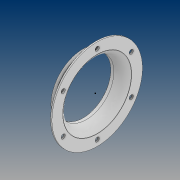
# Autodesk Inventor part: kelifos 3
Saved by Autodesk Inventor 2021 (Build 250183000, 183)
## iProperties
Created: 2021-01-08
Part Number: kelifos 3
Material: Generic
Document SubType Name: Sheet Metal
Designer: Διογενης Τσιχλακης
Density: 1 g/cm^3
Sheet Metal Rule: Default_mm
Appearance: Default
Author: Διογενης Τσιχλακης
Autodesk Inventor part; units mm, degrees
ref_plane "YZ Plane" through (0, 0, 0) normal (1, 0, 0) x (0, 1, 0)
ref_plane "XZ Plane" through (0, 0, 0) normal (0, 1, 0) x (-1, 0, 0)
ref_plane "XY Plane" through (0, 0, 0) normal (0, 0, 1) x (1, 0, 0)
sketch "Sketch1" plane through (0, 0, 0) normal (1, 0, 0) x (0, 1, 0)
  circle A0 centre (0, 0) radius 268
  circle A1 centre (0, 0) radius 232.5
  circle A2 centre (0, 0) radius 203.25
  circle A3 centre (232.5, 0) radius 12.5
  circle A4 centre (116.25, 201.3509) radius 12.5
  circle A5 centre (-116.25, 201.3509) radius 12.5
  circle A6 centre (-232.5, 0) radius 12.5
  circle A7 centre (-116.25, -201.3509) radius 12.5
  circle A8 centre (116.25, -201.3509) radius 12.5
  dimension "d1" = 465
  dimension "d0" = 536
  dimension "d2" = 406.5
  dimension "d3" = 25
  dimension "d52" = 360
  constraints: 8 centre point, 3 coincident, 1 horizontal alignment, 15 other
  measures "d0" diameter of A0
  measures "d2" diameter of A2
  measures "d3" diameter of A3
extrude "Extrusion1" add sketch "Sketch1" along normal blind 10 contours A0 | A3 A1 A8 A7 A6 A5 A4
sketch "Sketch2" plane through (0, 0, 0) normal (0, 1, 0) x (-1, 0, 0)
  line L0 (-10, 203.25) -> (0, 203.25) projected
  line L1 (-10, 203.25) -> (0, 203.25)
  line L2 (-10, 203.25) -> (-10, 193.1351)
  line L3 (-10, 188.8509) -> (-10, 213.8509) projected
  line L4 (0, 268) -> (0, -268) projected
  line L5 (0, 0) -> (70, 0)
  line L6 (70, 163.9189) -> (70, 0)
  line L7 (70, 0) -> (55, 0)
  line L8 (55, 163.9189) -> (55, 188.9189)
  line L9 (-10, -203.25) -> (-10, 203.25) projected
  line L10 (55, 163.9189) -> (55, 173.9189)
  line L11 (55, 188.9189) -> (65, 188.9189)
  line L12 (55, 163.9189) -> (65, 163.9189)
  line L13 (65, 163.9189) -> (70, 163.9189)
  line L14 (70, 188.9189) -> (65, 188.9189)
  line L15 (70, 163.9189) -> (75, 163.9189)
  line L16 (75, 163.9189) -> (75, 188.9189)
  line L17 (75, 188.9189) -> (70, 188.9189)
  line L18 (-10, 193.1351) -> (-10, 203.25)
  line L19 (-10, 268) -> (-10, -268) projected
  line L20 (55, 163.9189) -> (16.9075, 168.9189) construction
  line L21 (16.9075, 168.9189) -> (2.8778, 183.1289) construction
  line L22 (2.8778, 183.1289) -> (-3.4433, 190.5056) construction
  line L23 (-3.4433, 190.5056) -> (-10, 203.25) construction
  spline S0 degree 4 poles (55, 163.9189) (16.9075, 168.9189) (2.8778, 183.1289) (-3.4433, 190.5056) (-10, 203.25) knots 1 1 1 1 1 2 2 2 2 2
  line L24 (55, 172.7781) -> (24.3468, 173.9761) construction
  line L25 (24.3468, 173.9761) -> (10.3171, 188.1861) construction
  line L26 (10.3171, 188.1861) -> (3.996, 195.5628) construction
  line L27 (3.996, 195.5628) -> (-2.5607, 208.3073) construction
  spline S1 degree 4 poles (55, 172.7781) (24.3468, 173.9761) (10.3171, 188.1861) (3.996, 195.5628) (-2.5607, 208.3073) knots 1 1 1 1 1 2 2 2 2 2
  point P0 (0, 188.9189)
  point P1 (0, 203.6222)
  dimension "d43" = 163.9189
  dimension "d44" = 188.9189
  constraints: 30 end point, 5 horizontal, 5 point on line, 3 collinear, 2 perpendicular, 2 vertical, 6 other
  measures "d43" distance of L6.start L5.end
  measures "d44" distance between parallel lines of L5 L11
revolve "Revolution1" add sketch "Sketch2" angle 360 about axis through (0, 0, 0) along (-1, 0, 0) contours L0 L4 S0 | L4 S1 L8 S0 | L8 L11 L14 L17 L16 L15 L13 L12
sketch "Sketch4" plane through (0, 0, 0) normal (0, 1, 0) x (-1, 0, 0)
  point P0 (0, 0)
sketch "Sketch5" plane through (-75, 0, 0) normal (-1, 0, 0) x (0, 0, 1)
  circle A0 centre (0, 0) radius 176.5
  circle A1 centre (176.5, 0) radius 5
  dimension "d15" = 353
  dimension "d16" = 10
  constraints: 1 centre point, 1 coincident, 1 horizontal alignment, 2 other
  measures "d16" diameter of A1
extrude "Extrusion3" cut sketch "Sketch5" against normal blind 10 contours A0 A1 | A0 A1 picked at (174.9371, -1.1415) picked at (177.9961, -1.2848)
sketch "Sketch6" plane through (0, 0, 0) normal (0, 1, 0) x (-1, 0, 0)
  line L0 (65, 181.5) -> (65, 171.5) projected
  line L1 (65, 171.5) -> (65, 176.5)
  line L2 (65, 176.5) -> (60, 176.5)
  line L3 (60, 176.5) -> (65, 171.5)
  point P0 (0, 0)
  constraints: 6 end point, 1 collinear, 1 horizontal
revolve "Revolution2" cut sketch "Sketch6" angle 360 about axis through (-65, 0, 176.5) along (1, 0, 0)
thread "Thread1" size "M10x1.5" class "6H" standard "ANSI Metric M Profile" full length
pattern_circular "Circular Pattern1" count 8 over 360 about axis through (-65, 0, 0) along (-1, 0, 0) of "Revolution2", "Extrusion3"
thread "Thread2" size "M10x1.5" class "6H" standard "ANSI Metric M Profile" full length
thread "Thread3" size "M10x1.5" class "6H" standard "ANSI Metric M Profile" full length
thread "Thread4" size "M10x1.5" class "6H" standard "ANSI Metric M Profile" full length
thread "Thread5" size "M10x1.5" class "6H" standard "ANSI Metric M Profile" full length
thread "Thread6" size "M10x1.5" class "6H" standard "ANSI Metric M Profile" full length
thread "Thread7" size "M10x1.5" class "6H" standard "ANSI Metric M Profile" full length
thread "Thread8" size "M10x1.5" class "6H" standard "ANSI Metric M Profile" full length
thread "Thread9" size "M10x1.5" class "6H" standard "ANSI Metric M Profile" full length
fillet "Fillet2" radius 4 2 edges at (10, 0, -203.25) (0, 0, -203.6222)
fillet "Fillet3" radius 4 1 edges at (-55, 0, -172.7781)
fillet "Fillet4" radius 2 1 edges at (-75, 0, -163.9189)
fillet "Fillet5" radius 2 2 edges at (-55, 0, -188.9189) (0, -268, 0)
equation "\"BendRadius\" = Thickness"
equation "\"BendReliefWidth\" = Thickness"
equation "\"BendReliefDepth\" = 0.5 * Thickness"
equation "\"CornerReliefSize\" = 4 * Thickness"
equation "\"MinimumRemnant\" = 2 * Thickness"
equation "\"TransitionRadius\" = BendRadius"
equation "\"JacobiRadiusSize\" = BendRadius"
equation "\"GapSize\" = Thickness"
equation "\"Thickness\" = 0.5"
body "Solid1"
